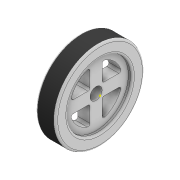
# Autodesk Inventor part: cock wheel
Saved by Autodesk Inventor 2021 (Build 250183000, 183)
## iProperties
Created: 2021-06-21
Part Number: cock wheel
Material: Generic
Document SubType Name: Modeling
Designer: user
Density: 1 g/cm^3
Appearance: Default
Author: user
Autodesk Inventor part; units mm, degrees
ref_plane "YZ Plane" through (0, 0, 0) normal (1, 0, 0) x (0, 1, 0)
ref_plane "XZ Plane" through (0, 0, 0) normal (0, 1, 0) x (-1, 0, 0)
ref_plane "XY Plane" through (0, 0, 0) normal (0, 0, 1) x (1, 0, 0)
sketch "Sketch1" plane through (0, 0, 0) normal (1, 0, 0) x (0, 1, 0)
  point P0 (0, 0)
sketch "Sketch2" plane through (0, 0, 0) normal (1, 0, 0) x (0, 1, 0)
  circle A0 centre (0, 0) radius 69.85
  dimension "d0" = 139.7
  constraints: 1 centre point, 1 coincident
  measures "d0" diameter of A0
extrude "Extrusion1" add sketch "Sketch2" along normal blind 31.75
sketch "Sketch3" plane through (0, 0, 0) normal (-1, 0, 0) x (0, 0, 1)
  circle A0 centre (0, 0) radius 50.8
  dimension "d3" = 101.6
  constraints: 1 centre point, 1 coincident
  measures "d3" diameter of A0
extrude "Extrusion2" cut sketch "Sketch3" against normal blind 6.35
sketch "Sketch4" plane through (31.75, 0, 0) normal (1, 0, 0) x (0, 0, -1)
  circle A0 centre (0, 0) radius 50.8
  dimension "d6" = 101.6
  constraints: 1 centre point, 1 coincident
  measures "d6" diameter of A0
extrude "Extrusion3" cut sketch "Sketch4" against normal blind 6.35
sketch "Sketch5" plane through (6.35, 0, 0) normal (-1, 0, 0) x (0, 0, 1)
  circle A0 centre (0, 0) radius 9.525
  line L0 (9.525, 0) -> (9.525, 40.1609)
  circle A1 centre (0, 0) radius 50.8 projected
  line L1 (9.525, -9.525) -> (9.525, -40.1609)
  line L2 (-9.525, 9.525) -> (-40.1609, 9.525)
  line L3 (9.525, 9.525) -> (40.1609, 9.525)
  line L4 (-9.525, 9.525) -> (-9.525, 40.1609)
  line L5 (-9.525, -9.525) -> (-9.525, -40.1609)
  line L6 (-9.525, -9.525) -> (-40.1609, -9.525)
  line L7 (9.525, -9.525) -> (40.1609, -9.525)
  arc A2 (9.525, -40.1609) -> (40.1609, -9.525) centre (0, 0) ccw
  arc A3 (40.1609, 9.525) -> (9.525, 40.1609) centre (0, 0) ccw
  arc A4 (-9.525, 40.1609) -> (-40.1609, 9.525) centre (0, 0) ccw
  arc A5 (-40.1609, -9.525) -> (-9.525, -40.1609) centre (0, 0) ccw
  constraints: 16 end point, 8 point on circle, 4 centre point, 3 horizontal, 3 vertical, 2 coincident, 2 perpendicular, 1 horizontal alignment, 1 point on line, 2 other
sketch "Sketch6" plane through (6.35, 0, 0) normal (-1, 0, 0) x (0, 0, 1)
  point P0 (0, 0)
sketch "Sketch7" plane through (6.35, 0, 0) normal (-1, 0, 0) x (0, 0, 1)
  point P0 (0, 0)
extrude "Extrusion4" cut sketch "Sketch5" against normal through all contours A0 | L0 A3 L3 | L7 A2 L1 | L2 A4 L4 | L5 A5 L6
fillet "Fillet1" radius 3.175 12 edges at (15.875, 9.525, -9.525) (15.875, 9.525, 9.525) (15.875, -9.525, 9.525) (15.875, 40.1609, 9.525) (15.875, 9.525, 40.1609) (15.875, -40.1609, 9.525) (15.875, 9.525, -40.1609) (15.875, -9.525, -9.525) (15.875, -9.525, -40.1609) (15.875, -40.1609, -9.525) (15.875, -9.525, 40.1609) (15.875, 40.1609, -9.525)
fillet "Fillet2" radius 3.175 4 edges at (0, -69.85, 0) (0, 0, -50.8) (31.75, -69.85, 0) (31.75, 0, 50.8)
sketch "Sketch8" plane through (31.75, 0, 0) normal (1, 0, 0) x (0, 0, -1)
  point P0 (0, 0)
sketch "Sketch9" plane through (0, 0, 0) normal (0, 1, 0) x (-1, 0, 0)
  point P0 (0, 0)
body "Solid1"
